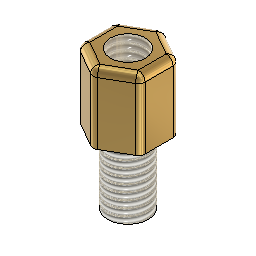
PCB Spacer M3x5mm (Autodesk Fusion 360 design; units mm, degrees)
Autodesk Fusion 360 part; units mm, degrees
sketch "Skizze1" plane through (0, 0, 0) normal (0, 0, 1) x (1, 0, 0)
  circle A0 centre (0, 0) radius 1.5
  line L0 (0, 0) -> (2.25, 0) construction
  line L1 (2.25, 1.299) -> (0, 2.5981)
  line L2 (0, 2.5981) -> (-2.25, 1.299)
  line L3 (-2.25, 1.299) -> (-2.25, -1.299)
  line L4 (-2.25, -1.299) -> (0, -2.5981)
  line L5 (0, -2.5981) -> (2.25, -1.299)
  line L6 (2.25, -1.299) -> (2.25, 1.299)
  dimension "d1" = 3
  dimension "d2" = 2.25
  constraint coincident A0.centre L0.start
  constraint horizontal L0
  measures "d1" diameter of A0
  measures "d2" distance of A0.centre L0.end
extrude "Extrusion1" add sketch "Skizze1" along normal blind 5 makes body 1
sketch "Skizze2" plane through (0, 0, 0) normal (0, 0, -1) x (1, 0, 0)
  circle A0 centre (0, 0) radius 1.5
  line L0 (2.25, -1.299) -> (2.25, 1.299)
  line L1 (2.25, 1.299) -> (0, 2.5981)
  line L2 (0, 2.5981) -> (-2.25, 1.299)
  line L3 (-2.25, 1.299) -> (-2.25, -1.299)
  line L4 (-2.25, -1.299) -> (0, -2.5981)
  line L5 (0, -2.5981) -> (2.25, -1.299)
  circle A1 centre (0, 0) radius 1.5
  dimension "d5" = 3
  constraint concentric A0 A1
  measures "d5" diameter of A1
extrude "Extrusion2" add sketch "Skizze2" along normal blind 5 separate body contours A0 A1 makes body 2
thread "Gewinde1" "ISO Metric profile 3.0 M3x0.5 6g" major diameter 2.927 minor diameter 2.3555 pitch 0.5 angle 60 resizes the face on face at (1.4981, 0.0748, -3.3333) on bodies 2
thread "Gewinde2" "ISO Metric profile 3.0 M3x0.5 6H" major diameter 3.086 minor diameter 2.529 pitch 0.5 angle 60 resizes the face on face at (1.4981, -0.0748, 3.3333) on bodies 1
fillet "Abrundung1" radius 0.5 1 edges at (1.125, 1.9486, 5) on bodies 1
fillet "Abrundung2" radius 0.5 3 edges at (0, 2.5981, 2.25) (-0.1464, 2.5135, 4.8536) (-1.375, 1.8042, 5) on bodies 1
fillet "Abrundung3" radius 0.5 3 edges at (-2.25, 1.299, 2.25) (-2.25, 1.1299, 4.8536) (-2.25, -0.2887, 5) on bodies 1
fillet "Abrundung4" radius 0.5 3 edges at (-2.25, -1.299, 2.25) (-2.1036, -1.3836, 4.8536) (-0.875, -2.0929, 5) on bodies 1
fillet "Abrundung5" radius 0.5 3 edges at (0, -2.5981, 2.25) (0.1464, -2.5135, 4.8536) (1.375, -1.8042, 5) on bodies 1
fillet "Abrundung6" radius 0.5 5 edges at (2.25, -1.299, 2.25) (2.25, -1.1299, 4.8536) (2.25, 0, 5) (2.25, 1.1299, 4.8536) (2.25, 1.299, 2.25) on bodies 1
